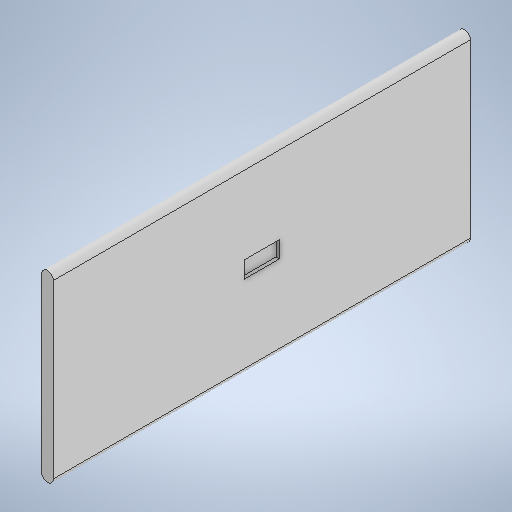
# Autodesk Inventor part: sensor
Saved by Autodesk Inventor 2025.2 (Build 292293000, 293)
## iProperties
Created: 2025-03-06
Part Number: sensor
Material: Genérico
Document SubType Name: Modeling
Designer: julia
Density: 1 g/cm^3
Appearance: Valor por defecto
Author: julia
Autodesk Inventor part; units mm, degrees
ref_plane "YZ Plane" through (0, 0, 0) normal (1, 0, 0) x (0, 1, 0)
ref_plane "XZ Plane" through (0, 0, 0) normal (0, 1, 0) x (-1, 0, 0)
ref_plane "XY Plane" through (0, 0, 0) normal (0, 0, 1) x (1, 0, 0)
sketch "Boceto1" plane through (0, 0, 0) normal (0, 0, 1) x (1, 0, 0)
  line L0 (0, 0) -> (0, 10.3) construction
  line L1 (0.35, 0) -> (0.35, 10.3)
  line L2 (-0.35, 10.3) -> (-0.35, 0)
  arc A0 (-0.35, 0) -> (0.35, 0) centre (0, 0) ccw
  arc A1 (0.35, 10.3) -> (-0.35, 10.3) centre (0, 10.3) ccw
  point P0 (0, 5.15)
  dimension "d0" = 10.3
  dimension "d1" = 0.7
  constraints: 8 end point, 4 point on circle, 4 tangent, 2 centre point, 1 midpoint, 1 parallel, 1 vertical
  measures "d0" distance of L0.start L0.end
  measures "d1" diameter of A1
extrude "Extrusión1" add sketch "Boceto1" along normal blind 25
sketch "Boceto2" plane through (0.35, 0, 0) normal (1, 0, 0) x (0, 0, -1)
  line L0 (-13.55, 4.65) -> (-11.45, 4.65)
  line L1 (-11.45, 4.65) -> (-11.45, 5.65)
  line L2 (-11.45, 5.65) -> (-13.55, 5.65)
  line L3 (-13.55, 5.65) -> (-13.55, 4.65)
  line L4 (-25, 0) -> (-25, 10.3) projected
  line L5 (0, 0) -> (-25, 0) projected
  point P0 (-12.5, 0)
  point P1 (-12.5, 4.65)
  dimension "d4" = 2.1
  dimension "d5" = 1
  dimension "d6" = 11.45
  dimension "d7" = 4.65
  constraints: 8 end point, 2 midpoint, 2 parallel, 1 horizontal, 1 perpendicular
  measures "d4" distance of L2.end L1.end
  measures "d5" distance of L1.end L0.end
  measures "d6" distance from line of L4 L0.start
  measures "d7" distance of point (-12.5, 0) point (-12.5, 4.65)
extrude "Extrusión2" cut sketch "Boceto2" against normal blind 0.2
